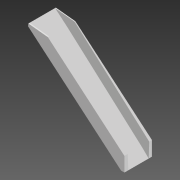
# Autodesk Inventor part: TopGrip
Saved by Autodesk Inventor 2020.4 (Build 244396010, 396A)
## iProperties
Created: 2022-11-11
Part Number: TopGrip
Material: Generic
Document SubType Name: Modeling
Designer: Val
Density: 1 g/cm^3
Appearance: Default
Author: Val
Autodesk Inventor part; units mm, degrees
ref_plane "YZ Plane" through (0, 0, 0) normal (1, 0, 0) x (0, 1, 0)
ref_plane "XZ Plane" through (0, 0, 0) normal (0, 1, 0) x (-1, 0, 0)
sketch "Sketch1" plane through (0, 0, 0) normal (0, 0, 1) x (1, 0, 0)
  line L0 (-381.58, -848.5343) -> (-381.58, -825.2737)
  line L1 (-381.58, -825.2737) -> (-505.1463, -721.0439)
  line L2 (-505.1463, -721.0439) -> (-536.6679, -717.7157)
  line L3 (-381.58, -848.5343) -> (-386.946, -848.5205)
  line L4 (-386.946, -848.5205) -> (-537.1054, -721.8591)
  line L5 (-537.1054, -721.8591) -> (-536.6679, -717.7157)
  line L6 (-381.58, -848.5343) -> (-536.6679, -717.7157) construction
  point P0 (0, 0)
  constraints: 12 end point, 1 perpendicular, 1 vertical
extrude "Extrusion1" add sketch "Sketch1" along normal mid plane 44.45
sketch "Sketch2" plane through (-505.1463, -721.0439, 22.225) normal (0.6447648, 0.764381, 0) x (0.764381, -0.6447648, 0)
  line L0 (0, 1.9422) -> (161.6554, 5.3274) projected
  line L1 (161.6554, 40.0134) -> (0, 43.18) projected
  line L2 (161.6554, 5.3274) -> (176.6531, 6.2699) projected
  line L3 (176.6531, 39.2056) -> (161.6554, 40.0134) projected
  line L4 (-26.2404, 2.0211) -> (0, 1.9422) projected
  line L5 (-26.2404, 43.18) -> (0, 43.18) projected
  line L6 (176.6531, 6.2699) -> (176.6531, 39.2056)
  line L7 (176.6531, 44.45) -> (176.6531, 0) projected
  line L8 (-26.2404, 2.0211) -> (-26.2404, 43.18)
  point P0 (-78.7795, 22.225)
  constraints: 4 end point, 1 collinear, 1 vertical
ref_plane "Work Plane1" through (-511.6606, -738.8097, -32.3222) normal (-0.6447648, -0.764381, 0) x (0.764381, -0.6447648, 0)
extrude "Extrusion2" cut sketch "Sketch2" against normal up to surface (17.78 mm away)
body "Solid1"
